e8f409db-14d5-41d7-b1c2-7f1d888f9dd6 (Autodesk Fusion 360 design; units mm, degrees)
Autodesk Fusion 360 part; units mm, degrees
sketch "Sketch2" plane through (0, 0, 0) normal (1, 0, 0) x (0, 1, 0)
  line L0 (0, 0) -> (11.1252, 0) construction
  line L1 (22.5298, 0) -> (11.1252, 0) construction
  circle A0 centre (16.8275, 0) radius 5.7023
  dimension "d1" = 11.1252
  dimension "d2" = 22.5298
  constraint coincident L0.start origin
  constraint horizontal L0
  constraint parallel L0 L1
  constraint midpoint L1 A0.centre
  constraint coincident L1.start A0
  measures "d1" distance of L0.start L0.end
  measures "d2" distance of L0.start L1.start
revolve "Revolve4" add sketch "Sketch2" angle 360 about axis through (0, 0, 1.75) along (0, 0, 1) makes body 1
ref_plane "WorkPlane1" through (-22.5298, 0, 0) normal (1, 0, 0) x (0, 1, 0)
ref_plane "WorkPlane2" through (47.3202, 0, 0) normal (1, 0, 0) x (0, 1, 0)
ref_plane "WorkPlane3" through (18.7452, 0, 0) normal (1, 0, 0) x (0, 1, 0)
sketch "Sketch6" plane through (18.7452, 0, 0) normal (1, 0, 0) x (0, 1, 0)
  circle A0 centre (0, 0) radius 3.9688
  dimension "d31" = 7.9375
  constraint coincident A0.centre origin
  measures "d31" diameter of A0
extrude "Extrude1" add sketch "Sketch6" along normal up to surface (28.575 mm away) separate body makes body 2
ref_plane "WorkPlane4" through (16.8275, 0, 0) normal (1, 0, 0) x (0, 1, 0)
sketch "Sketch7" plane through (0, 0, 0) normal (0, 0, 1) x (1, 0, 0)
  line L0 (16.8275, 0.75) -> (16.8275, 21.75)
  line L1 (0, 0) -> (76.2, 0) construction
  line L2 (16.8275, 18.7283) -> (16.8275, -25.4) construction
  line L3 (16.8275, 0) -> (28.7338, 0)
  line L4 (28.7337, 0) -> (28.7337, 7.0323)
  line L5 (16.8275, 0) -> (16.8275, 3.9688)
  line L6 (26.4749, 8.4709) -> (16.8275, 3.9687)
  arc A0 (28.7337, 7.0323) -> (26.4749, 8.4709) centre (27.1462, 7.0323) ccw
  point P0 (28.7337, 9.525)
  dimension "d40" = 11.9062
  dimension "d41" = 9.525
  dimension "d42" = 3.9688
  dimension "d43" = 1.5875
  constraint coincident L1.start origin
  constraint horizontal L1
  constraint coincident L0 L2.start
  constraint parallel L0 L2
  constraint coincident L2 L3.start
  constraint coincident L1 L3.start
  constraint perpendicular L2 L3
  constraint perpendicular L3 L4
  constraint perpendicular L3 L5
  constraint coincident P0 L4
  constraint coincident P0 L6
  constraint tangent L4 A0
  constraint tangent L6 A0
  measures "d40" distance of L3.start L4.start
  measures "d41" distance of L4.start P0
  measures "d42" distance of L3.start L5.end
  measures "d43" radius of A0
revolve "Revolve5" add sketch "Sketch7" angle 360 about axis through (0, 0, 0) along (1, 0, 0) bodies 1 2
thread "Thread2" "ANSI Unified Screw Threads 0.3125 5/16-18 UNC 3A" major diameter 7.8283 minor diameter 6.2586 pitch 1.4111 angle 60 modelled right hand crest width 0.2172 on face at (34.9292, 3.949, 0.3952) crest through (28.381, 3.9141, 0) on bodies 1
fillet "Fillet2" radius 1.5875 1 edges at (21.649, -6.2123, 0.284) on bodies 1
equation "d27 = -d2"
equation "d28 = 2.750 in"
equation "d30 = -1.125 in"
equation "EyeInner = d1"
equation "EyeOuter = d2"
equation "ThreadDia = d31"
equation "TotalLength = d28"
equation "ShankLength = d30"
equation "d39 = d1 + ( ( d2 - d1 ) ) / 2"
equation "d40 = d31 * 1.5"
equation "d41 = d31 * 1.2"
equation "d42 = d31 / 2"
equation "d43 = d31 * 0.2"
equation "d45 = d31 * 0.2"
